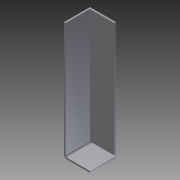
# Autodesk Inventor part: dozer side mid mount
Saved by Autodesk Inventor 2012 (Build 160160000, 160)
## iProperties
Created: 2013-10-07
Part Number: dozer side mid mount
Material: Default
Document SubType Name: Modeling
Designer: Bryce
Density: 1 g/cm^3
Author: Bryce
Autodesk Inventor part; units mm, degrees
ref_plane "YZ Plane" through (0, 0, 0) normal (1, 0, 0) x (0, 1, 0)
ref_plane "XZ Plane" through (0, 0, 0) normal (0, 1, 0) x (-1, 0, 0)
ref_plane "XY Plane" through (0, 0, 0) normal (0, 0, 1) x (1, 0, 0)
sketch "Sketch1" plane through (0, 0, 0) normal (0, 0, 1) x (1, 0, 0)
  line L0 (0, 0) -> (25.4, 0)
  line L1 (25.4, 114.3) -> (0, 114.3)
  line L2 (0, 114.3) -> (0, 0)
  line L3 (25.4, 1.5875) -> (1.5875, 1.5875)
  line L4 (1.5875, 1.5875) -> (1.5875, 114.3)
  line L5 (25.4, 2.6988) -> (3.175, 2.6987)
  arc A0 (3.175, 2.6987) -> (3.175, 1.5875) centre (3.175, 2.1431) ccw
  line L6 (25.4, 0) -> (25.4, 1.5875)
  line L7 (25.4, 2.6988) -> (25.4, 114.3)
  dimension "d0" = 25.4
  dimension "d1" = 114.3
  dimension "d2" = 1.5875
  dimension "d3" = 1.5875
  dimension "d4" = 1.1113
  dimension "d5" = 1.5875
  constraints: 16 end point, 5 perpendicular, 3 parallel, 2 point on circle, 2 point on line, 2 tangent, 1 centre point, 1 collinear, 1 horizontal
  measures "d0" distance of L0.start L0.end
  measures "d1" distance of L1.end L0.start
  measures "d2" distance between parallel lines of L0 L3
  measures "d3" distance between parallel lines of L2 L4
  measures "d4" distance between parallel lines of L3 L5
  measures "d5" distance from line of L4 A0.centre
extrude "Extrusion1" add sketch "Sketch1" along normal blind 25.4 contours L2 L1 L4 L3 L6 L0
extrude "Extrusion2" add sketch "Sketch1" along normal blind 1.5875 contours L1 L7 L5 A0 L3 L4
fillet "Fillet1" radius 1.5875 1 edges at (1.5875, 1.5875, 13.4938)
fillet "Fillet2" radius 3.175 1 edges at (0, 0, 12.7)
equation "\"d2\" = d3"
equation "\"d4\" = 0.7 * d2"
body "Solid1"
